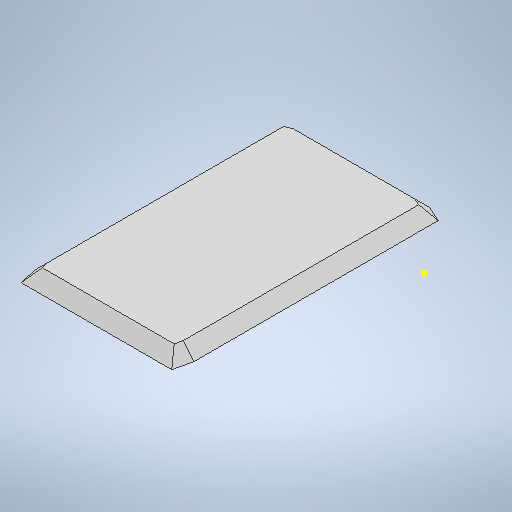
# Autodesk Inventor part: Part3edd
Saved by Autodesk Inventor 2025.2 (Build 292293000, 293)
## iProperties
Created: 2025-06-06
Part Number: Part3edd
Material: Generic
Document SubType Name: Sheet Metal
Designer: ziyuz
Density: 1 g/cm^3
Sheet Metal Rule: Default_mm
Appearance: Default
Author: ziyuz
Autodesk Inventor part; units mm, degrees
ref_plane "YZ Plane" through (0, 0, 0) normal (1, 0, 0) x (0, 1, 0)
ref_plane "XZ Plane" through (0, 0, 0) normal (0, 1, 0) x (-1, 0, 0)
ref_plane "XY Plane" through (0, 0, 0) normal (0, 0, 1) x (1, 0, 0)
sketch "Sketch1" plane through (0, 0, 0) normal (0, 1, 0) x (-1, 0, 0)
  line L0 (11.1472, -12.1394) -> (32.7528, -12.1394)
  line L1 (32.7528, -12.1394) -> (11.1472, -12.1394)
  line L2 (8.45, -10.938) -> (11.1472, -12.1394)
  line L3 (11.1472, -12.1394) -> (8.45, -10.938)
  line L4 (8.45, -10.938) -> (10.45, -9.6394)
  line L5 (8.45, 30.5881) -> (8.45, -10.938)
  line L6 (8.45, -10.938) -> (8.45, 30.5881)
  line L7 (9.1529, 33.6372) -> (10.7443, 31.6372)
  line L8 (8.45, 30.5881) -> (9.1529, 33.6372)
  line L9 (35.45, -10.938) -> (35.45, 30.5881)
  line L10 (8.45, -10.938) -> (35.45, -10.938)
  line L11 (35.45, 30.5881) -> (33.45, 30.3606)
  line L12 (8.45, 30.5881) -> (35.45, 30.5881)
  line L13 (34.747, 33.6372) -> (9.1529, 33.6372)
  line L14 (9.1529, 33.6372) -> (34.747, 33.6372)
  line L15 (11.1472, -12.1394) -> (32.7528, -12.1394)
  line L16 (8.45, 30.5881) -> (9.1529, 33.6372)
  line L17 (9.1529, 33.6372) -> (34.747, 33.6372)
  line L18 (11.5725, -10.1394) -> (32.3275, -10.1394)
  line L19 (32.3275, -10.1394) -> (11.5725, -10.1394)
  line L20 (11.1472, -12.1394) -> (8.45, -10.938)
  line L21 (8.45, -10.938) -> (8.45, 30.5881)
  line L22 (8.45, 30.5881) -> (9.1529, 33.6372)
  line L23 (34.747, 33.6372) -> (9.1529, 33.6372)
  line L24 (35.45, 30.5881) -> (34.747, 33.6372)
  line L25 (34.747, 33.6372) -> (35.45, 30.5881)
  line L26 (32.7528, -12.1394) -> (35.45, -10.938)
  line L27 (32.7528, -12.1394) -> (35.45, -10.938)
  line L28 (33.45, -9.6394) -> (33.45, 30.3606)
  line L29 (32.3275, -10.1394) -> (33.45, -9.6394)
  line L30 (33.45, 30.3606) -> (33.45, -9.6394)
  line L31 (32.3275, -10.1394) -> (11.5725, -10.1394)
  line L32 (10.45, -9.6394) -> (11.5725, -10.1394)
  line L33 (11.5725, -10.1394) -> (10.45, -9.6394)
  line L34 (10.45, -9.6394) -> (10.45, 30.3606)
  line L35 (10.45, 30.3606) -> (10.7443, 31.6372)
  line L36 (33.1557, 31.6372) -> (10.7443, 31.6372)
  line L37 (33.45, 30.3606) -> (33.1557, 31.6372)
  point P0 (0, 0)
  point P1 (-34.55, -34.6394)
  constraints: 76 end point, 9 collinear, 3 horizontal, 3 perpendicular, 3 vertical
extrude "Extrusion1" add sketch "Sketch1" along normal blind 2
chamfer "Chamfer1" distance 2 angle 45 8 edges at (-35.45, 2, 9.8251) (-35.0985, 2, 32.1127) (-21.95, 2, 33.6372) (-8.8014, 2, 32.1127) (-8.45, 2, 9.8251) (-21.95, 2, -12.1394) (-9.7986, 2, -11.5387) (-34.1014, 2, -11.5387)
sketch "Sketch2" plane through (0, 2, 0) normal (0, 1, 0) x (1, 0, 0)
  point P0 (0, 0)
equation "\"BendRadius\" = Thickness"
equation "\"BendReliefWidth\" = Thickness"
equation "\"BendReliefDepth\" = 0.5 * Thickness"
equation "\"CornerReliefSize\" = 4 * Thickness"
equation "\"MinimumRemnant\" = 2 * Thickness"
equation "\"TransitionRadius\" = BendRadius"
equation "\"JacobiRadiusSize\" = BendRadius"
equation "\"GapSize\" = Thickness"
equation "\"Thickness\" = 0.5"
body "Solid1"
